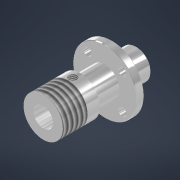
# Autodesk Inventor part: 022
Saved by Autodesk Inventor 2022 (Build 260153000, 153)
## iProperties
Created: 2021-11-20
Part Number: 022
Material: Aluminum 6061
Document SubType Name: Modeling
Designer: vinicius.miguel
Density: 2.7 g/cm^3
Appearance: Aluminum - Flat
Author: vinicius.miguel
Autodesk Inventor part; units mm, degrees
ref_plane "YZ Plane" through (0, 0, 0) normal (1, 0, 0) x (0, 1, 0)
ref_plane "XY Plane" through (0, 0, 0) normal (0, 0, 1) x (1, 0, 0)
sketch "Sketch1" plane through (0, 0, 0) normal (1, 0, 0) x (0, 1, 0)
  line L0 (0, 0) -> (0, 28)
  line L1 (6, -10) -> (6, 0)
  line L2 (6, 0) -> (13, 0)
  line L3 (13, 0) -> (13, 3)
  line L4 (13, 3) -> (6, 3)
  line L5 (6, 3) -> (6, 28)
  line L6 (6, 28) -> (4, 28)
  line L7 (6, -10) -> (4, -10)
  line L8 (4, -10) -> (4, -9)
  line L9 (4, -9) -> (4.75, -9)
  line L10 (4.75, -7.5) -> (4, -7.5)
  line L11 (4, -7.5) -> (4, 28)
  line L12 (6, 13) -> (8, 13)
  line L13 (8, 13) -> (8, 28)
  line L14 (8, 28) -> (6, 28)
  line L15 (4.75, -9) -> (4.75, -7.5)
  dimension "d1" = 8
  dimension "d2" = 12
  dimension "d4" = 1
  dimension "d5" = 26
  dimension "d6" = 3
  dimension "d7" = 25
  dimension "d8" = 10
  dimension "d21" = 10
  dimension "d22" = 16
  dimension "d37" = 1.5
  dimension "d38" = 0.75
  constraints: 32 end point, 8 perpendicular, 3 horizontal, 3 point on line, 3 vertical, 1 horizontal alignment, 1 parallel, 1 vertical alignment
  measures "d1" diameter of L11 L0
  measures "d2" diameter of L1 L0
  measures "d4" distance of L7.end L8.end
  measures "d5" diameter of L3 L0
  measures "d6" distance of L2.end L3.end
  measures "d7" distance of L4.end L5.end
  measures "d8" distance of L1.start L1.end
  measures "d21" distance between parallel lines of L12 L4
  measures "d22" diameter of L13 L0
  measures "d37" distance of L9.end L10.start
  measures "d38" distance of L10.start L10.end
revolve "Revolution1" add sketch "Sketch1" angle 360 about axis through (0, 0, 0) along (0, 0, 1)
sketch "Sketch2" plane through (0, 0, 3) normal (0, 0, 1) x (1, 0, 0)
  line L0 (0, 0) -> (7.0711, 7.0711)
  line L1 (0, 0) -> (0, 5.4649)
  dimension "d42" = 10
  dimension "d43" = 45
  constraints: 4 end point, 1 coincident, 1 vertical
  measures "d42" distance of L0.start L0.end
  measures "d43" angle of L0 L1
hole "Hole1" at (7.0711, 7.0711, 3) direction (0, 0, -1) diameter 3.4 end through all clearance for "Countersunk Flat Head Screw ISO 2009/7046" size "M3" standard "ISO"
pattern_circular "Circular Pattern1" count 4 over 360 about axis through (0, 0, 8) along (0, 0, -1) of "Hole1"
ref_plane "Work Plane1" through (0, 8, 20.5) normal (0, 1, 0) x (-1, 0, 0)
sketch "Sketch3" plane through (0, 8, 20.5) normal (0, 1, 0) x (-1, 0, 0)
  line L0 (-8, -7.5) -> (8, -7.5) projected
  point P0 (0, -20.5)
  point P1 (0, -4.5)
  point P2 (0, -7.5)
  dimension "d23" = 3
  constraints: 1 midpoint, 1 vertical alignment
  measures "d23" distance from line of point (0, -4.5) L0
hole "Hole2" at (0, 8, 16) direction (0, -1, 0) diameter 3.242 depth 10 thread size "M4x0.7" class "6H" standard "ISO Metric profile"
chamfer "Chamfer1" distance 0.5 angle 45 1 edges at (0, -6, -10)
thread "Thread1" size "M16x2" class "6g" standard "ANSI Metric M Profile" length 10
chamfer "Chamfer2" distance 0.25 angle 45 2 edges at (0, -13, 3) (0, -13, 0)
body "Solid1"
